Autodesk Inventor part; units mm, degrees
(part 3 of 3)
  dimension "d56" = 0.5
  constraints: 660 point on circle, 400 end point, 333 centre point, 3 coincident
  measures "d54" diameter of A330
  measures "d55" diameter of A331
  measures "d56" radial gap between concentric circles of A332 A331
extrude "Extrusion7" [suppressed]
chamfer "Chamfer1" [suppressed]
extrude "Extrusion4" [suppressed]
extrude "Extrusion5" add sketch "Sketch4" along normal blind 7.3 and the other way blind 2.8 from surface at 0 separate body contours A0 L0 A1 A2 A3 L1 A4 L2 A5 L3 A6 A7 A8 L4 A9 L5 A10 L6 A11 A12 A13 L7 A14 L8 A15 L9 A16 A17 A18 L10 A19 L11 A20 L12 A21 A22 A23 L13 A24 L14 A25 L15 A26 A27 A28 L16 A29 L17 A30 L18 A31 A32 A33 L19 A34 L20 A35 L21 A36 A37 A38 L22 A39 L23 A40 L24 A41 A42 A43 L25 A44 L26 A45 L27 A46 A47 A48 L28 A49 L29 A50 L30 A51 A52 A53 L31 A54 L32 A55 L33 A56 A57 A58 L34 A59 L35
extrude "Extrusion6" cut sketch "Sketch2" along normal through all both and the other way through all contours A1 bodies 2 1
extrude "Extrusion11" add sketch "HTD3M 33Teeth" along normal blind 3.75 and the other way blind 2.75 separate body contours A1 L0 A2 L1 A3 L2 A4 A5 A6 L3 A7 L4 A8 L5 A9 A10 A11 L6 A12 L7 A13 L8 A14 A15 A16 L9 A17 L10 A18 L11 A19 A20 A21 L12 A22 L13 A23 L14 A24 A25 A26 L15 A27 L16 A28 L17 A29 A30 A31 L18 A32 L19 A33 L20 A34 A35 A36 L21 A37 L22 A38 L23 A39 A40 A41 L24 A42 L25 A43 L26 A44 A45 A46 L27 A47 L28 A48 L29 A49 A50 A51 L30 A52 L31 A53 L32 A54 A55 A56 L33 A57 L34 A58 L35 A59 A60 A61 L36 A62 L37 A63 L38 A64 A65 A66 L39 A67 L40 A68 L41 A69 A70 A71 L42 A72 L43 A73 L44 A74 A75 A76 L45 A77 L46 A78 L47 A79 A80 A81 L48 A82 L49 A83 L50 A84 A85 A86 L51 A87 L52 A88 L53 A89 A90 A91 L54 A92 L55 A93 L56 A94 A95 A96 L57 A97 L58 A98 L59 A99 A100 A101 L60 A102 L61 A103 L62 A104 A105 A106 L63 A107 L64 A108 L65 A109 A110 A111 L66 A112 L67 A113 L68 A114 A115 A116 L69 A117 L70 A118 L71 A119 A120 A121 L72 A122 L73 A123 L74 A124 A125 A126 L75 A127 L76 A128 L77 A129 A130 A131 L78 A132 L79 A133 L80 A134 A135 A136 L81 A137 L82 A138 L83 A139 A140 A141 L84 A142 L85 A143 L86 A144 A145 A146 L87 A147 L88 A148 L89 A149 A150 A151 L90 A152 L91 A153 L92 A154 A155 A156 L93 A157 L94 A158 L95 A159 A160 A161 L96 A162 L97 A163 L98 A164 A0
sketch "HTD3M 10 Teeth" plane through (0, 0, -2.75) normal (0, 0, -1) x (-1, 0, 0)
  circle A0 centre (0, 0) radius 5
  line L0 (0.8939, 3.7122) -> (1.1141, 4.1058)
  arc A1 (1.3267, 4.19) -> (1.1141, 4.1058) centre (1.272, 4.0174) ccw
  arc A2 (1.3895, 4.1696) -> (1.3267, 4.19) centre (0, 0) ccw
  arc A3 (1.512, 3.9765) -> (1.3895, 4.1696) centre (1.3323, 3.9979) ccw
  line L1 (1.512, 3.9765) -> (1.4588, 3.5286)
  arc A4 (1.4588, 3.5286) -> (1.8604, 2.6099) centre (2.4429, 3.4117) ccw
  line L2 (1.8604, 2.6099) -> (1.9073, 2.5759)
  arc A5 (1.9073, 2.5759) -> (2.9051, 2.4778) centre (2.4898, 3.3776) ccw
  line L3 (2.9051, 2.4778) -> (3.3146, 2.6668)
  arc A6 (3.5361, 2.61) -> (3.3146, 2.6668) centre (3.3905, 2.5025) ccw
  arc A7 (3.5749, 2.5565) -> (3.5361, 2.61) centre (0, 0) ccw
  arc A8 (3.5606, 2.3283) -> (3.5749, 2.5565) centre (3.4277, 2.4512) ccw
  line L4 (3.5606, 2.3283) -> (3.2543, 1.9972)
  arc A9 (3.2543, 1.9972) -> (3.0392, 1.018) centre (3.9817, 1.3242) ccw
  line L5 (3.0392, 1.018) -> (3.0571, 0.9628)
  arc A10 (3.0571, 0.9628) -> (3.8067, 0.297) centre (3.9996, 1.2691) ccw
  line L6 (3.8067, 0.297) -> (4.2491, 0.2092)
  arc A11 (4.3949, 0.033) -> (4.2491, 0.2092) centre (4.2139, 0.0317) ccw
  arc A12 (4.3949, -0.033) -> (4.3949, 0.033) centre (0, 0) ccw
  arc A13 (4.2491, -0.2092) -> (4.3949, -0.033) centre (4.2139, -0.0317) ccw
  line L7 (4.2491, -0.2092) -> (3.8067, -0.297)
  arc A14 (3.8067, -0.297) -> (3.0571, -0.9628) centre (3.9996, -1.2691) ccw
  line L8 (3.0571, -0.9628) -> (3.0392, -1.018)
  arc A15 (3.0392, -1.018) -> (3.2543, -1.9972) centre (3.9817, -1.3242) ccw
  line L9 (3.2543, -1.9972) -> (3.5606, -2.3283)
  arc A16 (3.5749, -2.5565) -> (3.5606, -2.3283) centre (3.4277, -2.4512) ccw
  arc A17 (3.5361, -2.61) -> (3.5749, -2.5565) centre (0, 0) ccw
  arc A18 (3.3146, -2.6668) -> (3.5361, -2.61) centre (3.3905, -2.5025) ccw
  line L10 (3.3146, -2.6668) -> (2.9051, -2.4778)
  arc A19 (2.9051, -2.4778) -> (1.9073, -2.5759) centre (2.4898, -3.3776) ccw
  line L11 (1.9073, -2.5759) -> (1.8604, -2.6099)
  arc A20 (1.8604, -2.6099) -> (1.4588, -3.5286) centre (2.4429, -3.4117) ccw
  line L12 (1.4588, -3.5286) -> (1.512, -3.9765)
  arc A21 (1.3895, -4.1696) -> (1.512, -3.9765) centre (1.3323, -3.9979) ccw
  arc A22 (1.3267, -4.19) -> (1.3895, -4.1696) centre (0, 0) ccw
  arc A23 (1.1141, -4.1058) -> (1.3267, -4.19) centre (1.272, -4.0174) ccw
  line L13 (1.1141, -4.1058) -> (0.8939, -3.7122)
  arc A24 (0.8939, -3.7122) -> (0.029, -3.205) centre (0.029, -4.196) ccw
  line L14 (0.029, -3.205) -> (-0.029, -3.205)
  arc A25 (-0.029, -3.205) -> (-0.8939, -3.7122) centre (-0.029, -4.196) ccw
  line L15 (-0.8939, -3.7122) -> (-1.1141, -4.1058)
  arc A26 (-1.3267, -4.19) -> (-1.1141, -4.1058) centre (-1.272, -4.0174) ccw
  arc A27 (-1.3895, -4.1696) -> (-1.3267, -4.19) centre (0, 0) ccw
  arc A28 (-1.512, -3.9765) -> (-1.3895, -4.1696) centre (-1.3323, -3.9979) ccw
  line L16 (-1.512, -3.9765) -> (-1.4588, -3.5286)
  arc A29 (-1.4588, -3.5286) -> (-1.8604, -2.6099) centre (-2.4429, -3.4117) ccw
  line L17 (-1.8604, -2.6099) -> (-1.9073, -2.5759)
  arc A30 (-1.9073, -2.5759) -> (-2.9051, -2.4778) centre (-2.4898, -3.3776) ccw
  line L18 (-2.9051, -2.4778) -> (-3.3146, -2.6668)
  arc A31 (-3.5361, -2.61) -> (-3.3146, -2.6668) centre (-3.3905, -2.5025) ccw
  arc A32 (-3.5749, -2.5565) -> (-3.5361, -2.61) centre (0, 0) ccw
  arc A33 (-3.5606, -2.3283) -> (-3.5749, -2.5565) centre (-3.4277, -2.4512) ccw
  line L19 (-3.5606, -2.3283) -> (-3.2543, -1.9972)
  arc A34 (-3.2543, -1.9972) -> (-3.0392, -1.018) centre (-3.9817, -1.3242) ccw
  line L20 (-3.0392, -1.018) -> (-3.0571, -0.9628)
  arc A35 (-3.0571, -0.9628) -> (-3.8067, -0.297) centre (-3.9996, -1.2691) ccw
  line L21 (-3.8067, -0.297) -> (-4.2491, -0.2092)
  arc A36 (-4.3949, -0.033) -> (-4.2491, -0.2092) centre (-4.2139, -0.0317) ccw
  arc A37 (-4.3949, 0.033) -> (-4.3949, -0.033) centre (0, 0) ccw
  arc A38 (-4.2491, 0.2092) -> (-4.3949, 0.033) centre (-4.2139, 0.0317) ccw
  line L22 (-4.2491, 0.2092) -> (-3.8067, 0.297)
  arc A39 (-3.8067, 0.297) -> (-3.0571, 0.9628) centre (-3.9996, 1.2691) ccw
  line L23 (-3.0571, 0.9628) -> (-3.0392, 1.018)
  arc A40 (-3.0392, 1.018) -> (-3.2543, 1.9972) centre (-3.9817, 1.3242) ccw
  line L24 (-3.2543, 1.9972) -> (-3.5606, 2.3283)
  arc A41 (-3.5749, 2.5565) -> (-3.5606, 2.3283) centre (-3.4277, 2.4512) ccw
  arc A42 (-3.5361, 2.61) -> (-3.5749, 2.5565) centre (0, 0) ccw
  arc A43 (-3.3146, 2.6668) -> (-3.5361, 2.61) centre (-3.3905, 2.5025) ccw
  line L25 (-3.3146, 2.6668) -> (-2.9051, 2.4778)
  arc A44 (-2.9051, 2.4778) -> (-1.9073, 2.5759) centre (-2.4898, 3.3776) ccw
  line L26 (-1.9073, 2.5759) -> (-1.8604, 2.6099)
  arc A45 (-1.8604, 2.6099) -> (-1.4588, 3.5286) centre (-2.4429, 3.4117) ccw
  line L27 (-1.4588, 3.5286) -> (-1.512, 3.9765)
  arc A46 (-1.3895, 4.1696) -> (-1.512, 3.9765) centre (-1.3323, 3.9979) ccw
  arc A47 (-1.3267, 4.19) -> (-1.3895, 4.1696) centre (0, 0) ccw
  arc A48 (-1.1141, 4.1058) -> (-1.3267, 4.19) centre (-1.272, 4.0174) ccw
  line L28 (-1.1141, 4.1058) -> (-0.8939, 3.7122)
  arc A49 (-0.8939, 3.7122) -> (-0.029, 3.205) centre (-0.029, 4.196) ccw
  line L29 (-0.029, 3.205) -> (0.029, 3.205)
  arc A50 (0.029, 3.205) -> (0.8939, 3.7122) centre (0.029, 4.196) ccw
  circle A51 centre (0, 0) radius 6.9
  circle A52 centre (0, 0) radius 5.1866
  arc A53 (-0.029, -3.405) -> (-0.7193, -3.8098) centre (-0.029, -4.196) ccw
  line L30 (-0.029, -3.405) -> (0.029, -3.405)
  arc A54 (0.7193, -3.8098) -> (0.029, -3.405) centre (0.029, -4.196) ccw
  line L31 (0.7193, -3.8098) -> (0.9395, -4.2034)
  arc A55 (0.9395, -4.2034) -> (1.387, -4.3807) centre (1.272, -4.0174) ccw
  arc A56 (1.387, -4.3807) -> (1.4527, -4.3593) centre (0, 0) ccw
  arc A57 (1.4527, -4.3593) -> (1.7106, -3.9529) centre (1.3323, -3.9979) ccw
  line L32 (1.7106, -3.9529) -> (1.6574, -3.505)
  arc A58 (1.9779, -2.7717) -> (1.6574, -3.505) centre (2.4429, -3.4117) ccw
  line L33 (1.9779, -2.7717) -> (2.0249, -2.7377)
  arc A59 (2.8213, -2.6594) -> (2.0249, -2.7377) centre (2.4898, -3.3776) ccw
  line L34 (2.8213, -2.6594) -> (3.2308, -2.8484)
  arc A60 (3.2308, -2.8484) -> (3.697, -2.7287) centre (3.3905, -2.5025) ccw
  arc A61 (3.697, -2.7287) -> (3.7376, -2.6729) centre (0, 0) ccw
  arc A62 (3.7376, -2.6729) -> (3.7074, -2.1925) centre (3.4277, -2.4512) ccw
  line L35 (3.7074, -2.1925) -> (3.4011, -1.8614)
  arc A63 (3.2294, -1.0798) -> (3.4011, -1.8614) centre (3.9817, -1.3242) ccw
  line L36 (3.2294, -1.0798) -> (3.2473, -1.0246)
  arc A64 (3.8456, -0.4932) -> (3.2473, -1.0246) centre (3.9996, -1.2691) ccw
  line L37 (3.8456, -0.4932) -> (4.288, -0.4054)
  arc A65 (4.288, -0.4054) -> (4.5949, -0.0345) centre (4.2139, -0.0317) ccw
  arc A66 (4.5949, -0.0345) -> (4.5949, 0.0345) centre (0, 0) ccw
  arc A67 (4.5949, 0.0345) -> (4.288, 0.4054) centre (4.2139, 0.0317) ccw
  line L38 (4.288, 0.4054) -> (3.8456, 0.4932)
  arc A68 (3.2473, 1.0246) -> (3.8456, 0.4932) centre (3.9996, 1.2691) ccw
  line L39 (3.2473, 1.0246) -> (3.2294, 1.0798)
  arc A69 (3.4011, 1.8614) -> (3.2294, 1.0798) centre (3.9817, 1.3242) ccw
  line L40 (3.4011, 1.8614) -> (3.7074, 2.1925)
  arc A70 (3.7074, 2.1925) -> (3.7376, 2.6729) centre (3.4277, 2.4512) ccw
  arc A71 (3.7376, 2.6729) -> (3.697, 2.7287) centre (0, 0) ccw
  arc A72 (3.697, 2.7287) -> (3.2308, 2.8484) centre (3.3905, 2.5025) ccw
  line L41 (3.2308, 2.8484) -> (2.8213, 2.6594)
  arc A73 (2.0249, 2.7377) -> (2.8213, 2.6594) centre (2.4898, 3.3776) ccw
  line L42 (2.0249, 2.7377) -> (1.9779, 2.7717)
  arc A74 (1.6574, 3.505) -> (1.9779, 2.7717) centre (2.4429, 3.4117) ccw
  line L43 (1.6574, 3.505) -> (1.7106, 3.9529)
  arc A75 (1.7106, 3.9529) -> (1.4527, 4.3593) centre (1.3323, 3.9979) ccw
  arc A76 (1.4527, 4.3593) -> (1.387, 4.3807) centre (0, 0) ccw
  arc A77 (1.387, 4.3807) -> (0.9395, 4.2034) centre (1.272, 4.0174) ccw
  line L44 (0.9395, 4.2034) -> (0.7193, 3.8098)
  arc A78 (0.029, 3.405) -> (0.7193, 3.8098) centre (0.029, 4.196) ccw
  line L45 (0.029, 3.405) -> (-0.029, 3.405)
  arc A79 (-0.7193, 3.8098) -> (-0.029, 3.405) centre (-0.029, 4.196) ccw
  line L46 (-0.7193, 3.8098) -> (-0.9395, 4.2034)
  arc A80 (-0.9395, 4.2034) -> (-1.387, 4.3807) centre (-1.272, 4.0174) ccw
  arc A81 (-1.387, 4.3807) -> (-1.4527, 4.3593) centre (0, 0) ccw
  arc A82 (-1.4527, 4.3593) -> (-1.7106, 3.9529) centre (-1.3323, 3.9979) ccw
  line L47 (-1.7106, 3.9529) -> (-1.6574, 3.505)
  arc A83 (-1.9779, 2.7717) -> (-1.6574, 3.505) centre (-2.4429, 3.4117) ccw
  line L48 (-1.9779, 2.7717) -> (-2.0249, 2.7377)
  arc A84 (-2.8213, 2.6594) -> (-2.0249, 2.7377) centre (-2.4898, 3.3776) ccw
  line L49 (-2.8213, 2.6594) -> (-3.2308, 2.8484)
  arc A85 (-3.2308, 2.8484) -> (-3.697, 2.7287) centre (-3.3905, 2.5025) ccw
  arc A86 (-3.697, 2.7287) -> (-3.7376, 2.6729) centre (0, 0) ccw
  arc A87 (-3.7376, 2.6729) -> (-3.7074, 2.1925) centre (-3.4277, 2.4512) ccw
  line L50 (-3.7074, 2.1925) -> (-3.4011, 1.8614)
  arc A88 (-3.2294, 1.0798) -> (-3.4011, 1.8614) centre (-3.9817, 1.3242) ccw
  line L51 (-3.2294, 1.0798) -> (-3.2473, 1.0246)
  arc A89 (-3.8456, 0.4932) -> (-3.2473, 1.0246) centre (-3.9996, 1.2691) ccw
  line L52 (-3.8456, 0.4932) -> (-4.288, 0.4054)
  arc A90 (-4.288, 0.4054) -> (-4.5949, 0.0345) centre (-4.2139, 0.0317) ccw
  arc A91 (-4.5949, 0.0345) -> (-4.5949, -0.0345) centre (0, 0) ccw
  arc A92 (-4.5949, -0.0345) -> (-4.288, -0.4054) centre (-4.2139, -0.0317) ccw
  line L53 (-4.288, -0.4054) -> (-3.8456, -0.4932)
  arc A93 (-3.2473, -1.0246) -> (-3.8456, -0.4932) centre (-3.9996, -1.2691) ccw
  line L54 (-3.2473, -1.0246) -> (-3.2294, -1.0798)
  arc A94 (-3.4011, -1.8614) -> (-3.2294, -1.0798) centre (-3.9817, -1.3242) ccw
  line L55 (-3.4011, -1.8614) -> (-3.7074, -2.1925)
  arc A95 (-3.7074, -2.1925) -> (-3.7376, -2.6729) centre (-3.4277, -2.4512) ccw
  arc A96 (-3.7376, -2.6729) -> (-3.697, -2.7287) centre (0, 0) ccw
  arc A97 (-3.697, -2.7287) -> (-3.2308, -2.8484) centre (-3.3905, -2.5025) ccw
  line L56 (-3.2308, -2.8484) -> (-2.8213, -2.6594)
  arc A98 (-2.0249, -2.7377) -> (-2.8213, -2.6594) centre (-2.4898, -3.3776) ccw
  line L57 (-2.0249, -2.7377) -> (-1.9779, -2.7717)
  arc A99 (-1.6574, -3.505) -> (-1.9779, -2.7717) centre (-2.4429, -3.4117) ccw
  line L58 (-1.6574, -3.505) -> (-1.7106, -3.9529)
  arc A100 (-1.7106, -3.9529) -> (-1.4527, -4.3593) centre (-1.3323, -3.9979) ccw
  arc A101 (-1.4527, -4.3593) -> (-1.387, -4.3807) centre (0, 0) ccw
  arc A102 (-1.387, -4.3807) -> (-0.9395, -4.2034) centre (-1.272, -4.0174) ccw
  line L59 (-0.9395, -4.2034) -> (-0.7193, -3.8098)
  circle A103 centre (0, 0) radius 2.075
  arc A104 (-0.029, -3.455) -> (-0.6757, -3.8342) centre (-0.029, -4.196) ccw
  line L60 (-0.029, -3.455) -> (0.029, -3.455)
  arc A105 (0.6757, -3.8342) -> (0.029, -3.455) centre (0.029, -4.196) ccw
  line L61 (0.6757, -3.8342) -> (0.8959, -4.2279)
  arc A106 (0.8959, -4.2279) -> (1.4021, -4.4283) centre (1.272, -4.0174) ccw
  arc A107 (1.4021, -4.4283) -> (1.4685, -4.4067) centre (0, 0) ccw
  arc A108 (1.4685, -4.4067) -> (1.7603, -3.947) centre (1.3323, -3.9979) ccw
  line L62 (1.7603, -3.947) -> (1.7071, -3.4991)
  arc A109 (2.0073, -2.8122) -> (1.7071, -3.4991) centre (2.4429, -3.4117) ccw
  line L63 (2.0073, -2.8122) -> (2.0543, -2.7781)
  arc A110 (2.8003, -2.7048) -> (2.0543, -2.7781) centre (2.4898, -3.3776) ccw
  line L64 (2.8003, -2.7048) -> (3.2099, -2.8938)
  arc A111 (3.2099, -2.8938) -> (3.7373, -2.7584) centre (3.3905, -2.5025) ccw
  arc A112 (3.7373, -2.7584) -> (3.7783, -2.7019) centre (0, 0) ccw
  arc A113 (3.7783, -2.7019) -> (3.7441, -2.1585) centre (3.4277, -2.4512) ccw
  line L65 (3.7441, -2.1585) -> (3.4378, -1.8274)
  arc A114 (3.2769, -1.0952) -> (3.4378, -1.8274) centre (3.9817, -1.3242) ccw
  line L66 (3.2769, -1.0952) -> (3.2949, -1.0401)
  arc A115 (3.8554, -0.5422) -> (3.2949, -1.0401) centre (3.9996, -1.2691) ccw
  line L67 (3.8554, -0.5422) -> (4.2978, -0.4544)
  arc A116 (4.2978, -0.4544) -> (4.6449, -0.0349) centre (4.2139, -0.0317) ccw
  arc A117 (4.6449, -0.0349) -> (4.6449, 0.0349) centre (0, 0) ccw
  arc A118 (4.6449, 0.0349) -> (4.2978, 0.4544) centre (4.2139, 0.0317) ccw
  line L68 (4.2978, 0.4544) -> (3.8554, 0.5422)
  arc A119 (3.2949, 1.0401) -> (3.8554, 0.5422) centre (3.9996, 1.2691) ccw
  line L69 (3.2949, 1.0401) -> (3.2769, 1.0952)
  arc A120 (3.4378, 1.8274) -> (3.2769, 1.0952) centre (3.9817, 1.3242) ccw
  line L70 (3.4378, 1.8274) -> (3.7441, 2.1585)
  arc A121 (3.7441, 2.1585) -> (3.7783, 2.7019) centre (3.4277, 2.4512) ccw
  arc A122 (3.7783, 2.7019) -> (3.7373, 2.7584) centre (0, 0) ccw
  arc A123 (3.7373, 2.7584) -> (3.2099, 2.8938) centre (3.3905, 2.5025) ccw
  line L71 (3.2099, 2.8938) -> (2.8003, 2.7048)
  arc A124 (2.0543, 2.7781) -> (2.8003, 2.7048) centre (2.4898, 3.3776) ccw
  line L72 (2.0543, 2.7781) -> (2.0073, 2.8122)
  arc A125 (1.7071, 3.4991) -> (2.0073, 2.8122) centre (2.4429, 3.4117) ccw
  line L73 (1.7071, 3.4991) -> (1.7603, 3.947)
  arc A126 (1.7603, 3.947) -> (1.4685, 4.4067) centre (1.3323, 3.9979) ccw
  arc A127 (1.4685, 4.4067) -> (1.4021, 4.4283) centre (0, 0) ccw
  arc A128 (1.4021, 4.4283) -> (0.8959, 4.2279) centre (1.272, 4.0174) ccw
  line L74 (0.8959, 4.2279) -> (0.6757, 3.8342)
  arc A129 (0.029, 3.455) -> (0.6757, 3.8342) centre (0.029, 4.196) ccw
  line L75 (0.029, 3.455) -> (-0.029, 3.455)
  arc A130 (-0.6757, 3.8342) -> (-0.029, 3.455) centre (-0.029, 4.196) ccw
  line L76 (-0.6757, 3.8342) -> (-0.8959, 4.2279)
  arc A131 (-0.8959, 4.2279) -> (-1.4021, 4.4283) centre (-1.272, 4.0174) ccw
  arc A132 (-1.4021, 4.4283) -> (-1.4685, 4.4067) centre (0, 0) ccw
  arc A133 (-1.4685, 4.4067) -> (-1.7603, 3.947) centre (-1.3323, 3.9979) ccw
  line L77 (-1.7603, 3.947) -> (-1.7071, 3.4991)
  arc A134 (-2.0073, 2.8122) -> (-1.7071, 3.4991) centre (-2.4429, 3.4117) ccw
  line L78 (-2.0073, 2.8122) -> (-2.0543, 2.7781)
  arc A135 (-2.8003, 2.7048) -> (-2.0543, 2.7781) centre (-2.4898, 3.3776) ccw
  line L79 (-2.8003, 2.7048) -> (-3.2099, 2.8938)
  arc A136 (-3.2099, 2.8938) -> (-3.7373, 2.7584) centre (-3.3905, 2.5025) ccw
  arc A137 (-3.7373, 2.7584) -> (-3.7783, 2.7019) centre (0, 0) ccw
  arc A138 (-3.7783, 2.7019) -> (-3.7441, 2.1585) centre (-3.4277, 2.4512) ccw
  line L80 (-3.7441, 2.1585) -> (-3.4378, 1.8274)
  arc A139 (-3.2769, 1.0952) -> (-3.4378, 1.8274) centre (-3.9817, 1.3242) ccw
  line L81 (-3.2769, 1.0952) -> (-3.2949, 1.0401)
  arc A140 (-3.8554, 0.5422) -> (-3.2949, 1.0401) centre (-3.9996, 1.2691) ccw
  line L82 (-3.8554, 0.5422) -> (-4.2978, 0.4544)
  arc A141 (-4.2978, 0.4544) -> (-4.6449, 0.0349) centre (-4.2139, 0.0317) ccw
  arc A142 (-4.6449, 0.0349) -> (-4.6449, -0.0349) centre (0, 0) ccw
  arc A143 (-4.6449, -0.0349) -> (-4.2978, -0.4544) centre (-4.2139, -0.0317) ccw
  line L83 (-4.2978, -0.4544) -> (-3.8554, -0.5422)
  arc A144 (-3.2949, -1.0401) -> (-3.8554, -0.5422) centre (-3.9996, -1.2691) ccw
  line L84 (-3.2949, -1.0401) -> (-3.2769, -1.0952)
  arc A145 (-3.4378, -1.8274) -> (-3.2769, -1.0952) centre (-3.9817, -1.3242) ccw
  line L85 (-3.4378, -1.8274) -> (-3.7441, -2.1585)
  arc A146 (-3.7441, -2.1585) -> (-3.7783, -2.7019) centre (-3.4277, -2.4512) ccw
  arc A147 (-3.7783, -2.7019) -> (-3.7373, -2.7584) centre (0, 0) ccw
  arc A148 (-3.7373, -2.7584) -> (-3.2099, -2.8938) centre (-3.3905, -2.5025) ccw
  line L86 (-3.2099, -2.8938) -> (-2.8003, -2.7048)
  arc A149 (-2.0543, -2.7781) -> (-2.8003, -2.7048) centre (-2.4898, -3.3776) ccw
  line L87 (-2.0543, -2.7781) -> (-2.0073, -2.8122)
  arc A150 (-1.7071, -3.4991) -> (-2.0073, -2.8122) centre (-2.4429, -3.4117) ccw
  line L88 (-1.7071, -3.4991) -> (-1.7603, -3.947)
  arc A151 (-1.7603, -3.947) -> (-1.4685, -4.4067) centre (-1.3323, -3.9979) ccw
  arc A152 (-1.4685, -4.4067) -> (-1.4021, -4.4283) centre (0, 0) ccw
  arc A153 (-1.4021, -4.4283) -> (-0.8959, -4.2279) centre (-1.272, -4.0174) ccw
  line L89 (-0.8959, -4.2279) -> (-0.6757, -3.8342)
  point P0 (0, 0)
  dimension "d66" = 0.2
  dimension "d67" = 13.8
  dimension "d83" = 4.15
  dimension "d84" = 0.25
  constraints: 300 point on circle, 180 end point, 154 centre point, 2 coincident, 158 other
  measures "d66" radial gap between concentric circles of A25 A53
  measures "d67" diameter of A51
  measures "d83" diameter of A103
  measures "d84" radial gap between concentric circles of A25 A104
extrude "Extrusion15" add sketch "HTD3M 10 Teeth" along normal blind 2 contours A0 | A51 | A52 bodies 1
chamfer "Chamfer5" distance 2.2 distance2 1 1 edges at (6.9, 0, -4.75) measured on face at (6.4, 0, -4.75)
extrude "Extrusion16" cut sketch "HTD3M 10 Teeth" against normal blind 3 contours L0 A1 A2 A3 L1 A4 L2 A5 L3 A6 A7 A8 L4 A9 L5 A10 L6 A11 A12 A13 L7 A14 L8 A15 L9 A16 A17 A18 L10 A19 L11 A20 L12 A21 A22 A23 L13 A24 L14 A25 L15 A26 A27 A28 L16 A29 L17 A30 L18 A31 A32 A33 L19 A34 L20 A35 L21 A36 A37 A38 L22 A39 L23 A40 L24 A41 A42 A43 L25 A44 L26 A45 L27 A46 A47 A48 L28 A49 L29 A50 | A53 L59 A102 A101 A100 L58 A99 L57 A98 L56 A97 A96 A95 L55 A94 L54 A93 L53 A92 A91 A90 L52 A89 L51 A88 L50 A87 A86 A85 L49 A84 L48 A83 L47 A82 A81 A80 L46 A79 L45 A78 L44 A77 A76 A75 L43 A74 L42 A73 L41 A72 A71 A70 L40 A69 L39 A68 L38 A67 A66 A65 L37 A64 L36 A63 L35 A62 A61 A60 L34 A59 L33 A58 L32 A57 A56 A55 L31 A54 L30 | A104 L89 A153 A152 A151 L88 A150 L87 A149 L86 A148 A147 A146 L85 A145 L84 A144 L83 A143 A142 A141 L82 A140 L81 A139 L80 A138 A137 A136 L79 A135 L78 A134 L77 A133 A132 A131 L76 A130 L75 A129 L74 A128 A127 A126 L73 A125 L72 A124 L71 A123 A122 A121 L70 A120 L69 A119 L68 A118 A117 A116 L67 A115 L66 A114 L65 A113 A112 A111 L64 A110 L63 A109 L62 A108 A107 A106 L61 A105 L60 bodies 1
extrude "Extrusion12" add sketch "HTD3M 33Teeth" against normal blind 1.75 from surface at 3.75 contours A1 L0 A2 L1 A3 L2 A4 A5 A6 L3 A7 L4 A8 L5 A9 A10 A11 L6 A12 L7 A13 L8 A14 A15 A16 L9 A17 L10 A18 L11 A19 A20 A21 L12 A22 L13 A23 L14 A24 A25 A26 L15 A27 L16 A28 L17 A29 A30 A31 L18 A32 L19 A33 L20 A34 A35 A36 L21 A37 L22 A38 L23 A39 A40 A41 L24 A42 L25 A43 L26 A44 A45 A46 L27 A47 L28 A48 L29 A49 A50 A51 L30 A52 L31 A53 L32 A54 A55 A56 L33 A57 L34 A58 L35 A59 A60 A61 L36 A62 L37 A63 L38 A64 A65 A66 L39 A67 L40 A68 L41 A69 A70 A71 L42 A72 L43 A73 L44 A74 A75 A76 L45 A77 L46 A78 L47 A79 A80 A81 L48 A82 L49 A83 L50 A84 A85 A86 L51 A87 L52 A88 L53 A89 A90 A91 L54 A92 L55 A93 L56 A94 A95 A96 L57 A97 L58 A98 L59 A99 A100 A101 L60 A102 L61 A103 L62 A104 A105 A106 L63 A107 L64 A108 L65 A109 A110 A111 L66 A112 L67 A113 L68 A114 A115 A116 L69 A117 L70 A118 L71 A119 A120 A121 L72 A122 L73 A123 L74 A124 A125 A126 L75 A127 L76 A128 L77 A129 A130 A131 L78 A132 L79 A133 L80 A134 A135 A136 L81 A137 L82 A138 L83 A139 A140 A141 L84 A142 L85 A143 L86 A144 A145 A146 L87 A147 L88 A148 L89 A149 A150 A151 L90 A152 L91 A153 L92 A154 A155 A156 L93 A157 L94 A158 L95 A159 A160 A161 L96 A162 L97 A163 L98 A164 A0 | A331 | A332 bodies 3
chamfer "Chamfer4" distance 0.3 distance2 0.8 1 edges at (-16.25, 0, 2) measured on face at (-16.25, 0, 2.5)
extrude "Extrusion13" cut sketch "HTD3M 10 Teeth" against normal blind 1.75 contours L0 A1 A2 A3 L1 A4 L2 A5 L3 A6 A7 A8 L4 A9 L5 A10 L6 A11 A12 A13 L7 A14 L8 A15 L9 A16 A17 A18 L10 A19 L11 A20 L12 A21 A22 A23 L13 A24 L14 A25 L15 A26 A27 A28 L16 A29 L17 A30 L18 A31 A32 A33 L19 A34 L20 A35 L21 A36 A37 A38 L22 A39 L23 A40 L24 A41 A42 A43 L25 A44 L26 A45 L27 A46 A47 A48 L28 A49 L29 A50 | A53 L59 A102 A101 A100 L58 A99 L57 A98 L56 A97 A96 A95 L55 A94 L54 A93 L53 A92 A91 A90 L52 A89 L51 A88 L50 A87 A86 A85 L49 A84 L48 A83 L47 A82 A81 A80 L46 A79 L45 A78 L44 A77 A76 A75 L43 A74 L42 A73 L41 A72 A71 A70 L40 A69 L39 A68 L38 A67 A66 A65 L37 A64 L36 A63 L35 A62 A61 A60 L34 A59 L33 A58 L32 A57 A56 A55 L31 A54 L30 | A103 bodies 3
extrude "Extrusion14" add sketch "HTD3M 10 Teeth" along normal blind 7.3 and the other way blind 1.75 separate body contours L0 A1 A2 A3 L1 A4 L2 A5 L3 A6 A7 A8 L4 A9 L5 A10 L6 A11 A12 A13 L7 A14 L8 A15 L9 A16 A17 A18 L10 A19 L11 A20 L12 A21 A22 A23 L13 A24 L14 A25 L15 A26 A27 A28 L16 A29 L17 A30 L18 A31 A32 A33 L19 A34 L20 A35 L21 A36 A37 A38 L22 A39 L23 A40 L24 A41 A42 A43 L25 A44 L26 A45 L27 A46 A47 A48 L28 A49 L29 A50
equation "\"d1\" = da_a"
equation "\"d2\" = da_hg"
equation "\"d3\" = 2 * da_fi"
equation "\"d4\" = da_bw"
equation "\"d5\" = da_bf"
equation "\"d7\" = da_bf"
equation "\"d9\" = da_rb"
equation "\"d10\" = da_rt"
equation "\"da_pb\" = 2.5"
equation "\"da_fi\" = 25deg"
equation "\"da_hg\" = 0.75"
equation "\"da_bw\" = 1.05"
equation "\"da_rb\" = 0.2"
equation "\"da_rt\" = 0.3"
equation "\"da_a\" = 0.3"
equation "\"da_bf\" = 5.5"
equation "\"da_wf\" = 0.8"
equation "\"da_hf\" = 0.8"
